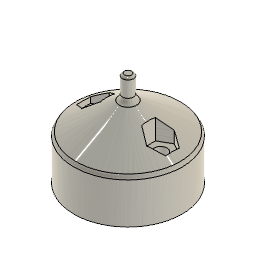
Cono de conexion v3 (Autodesk Fusion 360 design; units mm, degrees)
Autodesk Fusion 360 part; units mm, degrees
sketch "Boceto1" plane through (0, 0, 0) normal (0, 0, 1) x (1, 0, 0)
  circle A0 centre (0, 0) radius 12.5
  line L0 (12.5, 0) -> (-12.5, 0) construction
  circle A1 centre (0, 0) radius 4 construction
  circle A2 centre (0, 0) radius 2 construction
  circle A3 centre (7.5, 0) radius 1.5
  circle A4 centre (-7.5, 0) radius 1.5
  line L1 (7.5, -3.1754) -> (10.25, -1.5877)
  line L2 (10.25, -1.5877) -> (10.25, 1.5877)
  line L3 (10.25, 1.5877) -> (7.5, 3.1754)
  line L4 (7.5, 3.1754) -> (4.75, 1.5877)
  line L5 (4.75, 1.5877) -> (4.75, -1.5877)
  line L6 (4.75, -1.5877) -> (7.5, -3.1754)
  line L7 (-7.5, -3.1754) -> (-4.75, -1.5877)
  line L8 (-4.75, -1.5877) -> (-4.75, 1.5877)
  line L9 (-4.75, 1.5877) -> (-7.5, 3.1754)
  line L10 (-7.5, 3.1754) -> (-10.25, 1.5877)
  line L11 (-10.25, 1.5877) -> (-10.25, -1.5877)
  line L12 (-10.25, -1.5877) -> (-7.5, -3.1754)
  point P0 (7.5, 0)
  point P1 (-7.5, 0)
  dimension "d1" = 25
  dimension "d9" = 8
  dimension "d10" = 4
  dimension "d11" = 3
  dimension "d12" = 3
  dimension "d13" = 2.75
  dimension "d14" = 2.75
  dimension "d29" = 7.5
  dimension "d30" = 7.5
  constraint coincident A0.centre A1.centre
  constraint coincident A0 L0.start
  constraint coincident A0 L0.end
  constraint horizontal L0
  constraint concentric A1 A2
  constraint coincident L0 P0
  constraint coincident L0 P1
  constraint coincident P0 A3.centre
  constraint coincident P1 A4.centre
  constraint perpendicular L0 L11
  constraint perpendicular L0 L5
  measures "d1" diameter of A0
  measures "d9" diameter of A1
  measures "d10" diameter of A2
  measures "d11" diameter of A3
  measures "d12" diameter of A4
  measures "d13" distance of P0 L6
  measures "d14" distance of P1 L12
  measures "d29" distance of A0.centre P1
  measures "d30" distance of A0.centre P0
extrude "Extruir1" add sketch "Boceto1" against normal blind 10 contours A0 | A3 | A4 | L1 L2 L3 L4 L5 L6 | L7 L8 L9 L10 L11 L12
ref_plane "PlanoDeObra1" through (0, 0, 7) normal (0, 0, 1) x (1, 0, 0)
sketch "Boceto2" plane through (0, 0, 7) normal (0, 0, 1) x (1, 0, 0)
  circle A0 centre (0, 0) radius 12.5
  circle A1 centre (0, 0) radius 1.3
  dimension "d5" = -11.2
loft "Solevación1" add profiles "Boceto2" section 1 contours A1 section 2 face at (-3.3879, -0.621, 0)
sketch "Boceto3" plane through (0, 0, 7) normal (0, 0, 1) x (-1, 0, 0)
  circle A0 centre (0, 0) radius 1.3
  circle A1 centre (0, 0) radius 2
  dimension "d6" = 4
  constraint coincident A0.centre A1.centre
  measures "d6" diameter of A1
sketch "Boceto4" plane through (0, 0, 7) normal (0, 0, 1) x (-1, 0, 0)
  circle A0 centre (0, 0) radius 1.3
extrude "Extruir5" cut sketch "Boceto1" along normal blind 14 contours L1 L2 L3 L4 L5 L6
extrude "Extruir6" cut sketch "Boceto1" along normal blind 29 contours A3
extrude "Extruir7" cut sketch "Boceto1" along normal mid plane 60 contours A3
extrude "Extruir8" cut sketch "Boceto1" along normal blind 25 contours L7 L8 L9 L10 L11 L12
extrude "Extruir9" cut sketch "Boceto1" along normal mid plane 52 contours A4
extrude "Extruir11" add 1 faces at (-0.3369, 0.5261, 7) along direction (0, 0, 1) blind 5
fillet "Empalme1" radius 1.5 1 edges at (-1.212, 0.4701, 7)
fillet "Empalme2" radius 0.5 1 edges at (-1.212, -0.4701, 12)
fillet "Empalme3" radius 1 1 edges at (-11.6541, -4.5202, 0)
